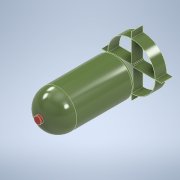
# Autodesk Inventor part: bomb
Saved by Autodesk Inventor 2022 (Build 260153000, 153)
## iProperties
Created: 2021-12-16
Part Number: bomb
Material: Generic
Document SubType Name: Modeling
Designer: jpc
Density: 1 g/cm^3
Appearance: Dark Olive
Author: jpc
Autodesk Inventor part; units mm, degrees
ref_plane "YZ Plane" through (0, 0, 0) normal (1, 0, 0) x (0, 1, 0)
ref_plane "XZ Plane" through (0, 0, 0) normal (0, 1, 0) x (-1, 0, 0)
ref_plane "XY Plane" through (0, 0, 0) normal (0, 0, 1) x (1, 0, 0)
sketch "Sketch1" plane through (0, 0, 0) normal (1, 0, 0) x (0, 1, 0)
  arc A0 (0, 250) -> (40, 251.6026) centre (0, 750) ccw
  line L0 (500, 750) -> (40, 750) construction
  line L1 (0, 750) -> (0, 250)
  line L2 (0, -750) -> (40, -750)
  line L3 (500, -750) -> (500, 750)
  line L4 (0, -750) -> (40, -750)
  line L5 (40, -750) -> (40, -1210) construction
  line L6 (40, -1500) -> (0, -1500)
  line L7 (0, -1500) -> (0, -750)
  line L8 (500, -750) -> (40, -1210)
  arc A1 (500, 750) -> (0, 1250) centre (0, 750) ccw
  arc A2 (0, 1250) -> (0, 250) centre (0, 750) ccw construction
  arc A3 (40, 251.6026) -> (500, 750) centre (0, 750) ccw construction
  line L9 (0, 250) -> (0, -750)
  line L10 (40, 750) -> (0, 750)
  line L11 (40, -750) -> (500, -750) construction
  line L12 (40, -1210) -> (40, -1500)
  line L13 (0, 1250) -> (0, 750)
  line L14 (500, 0) -> (0, 0)
  dimension "d1" = 1500
  dimension "d2" = 750
  dimension "d3" = 40
  dimension "d4" = 45
  dimension "d6" = 1000
  constraints: 30 end point, 9 parallel, 8 point on circle, 7 perpendicular, 4 centre point, 4 point on line, 3 horizontal, 2 coincident, 1 collinear, 1 midpoint
  measures "d1" distance of L3.start L0.start
  measures "d2" distance of L2.end L6.start
  measures "d3" distance of L6.start L6.end
  measures "d4" angle of L5 L8
  measures "d6" diameter of L3 L9
revolve "Revolution1" add sketch "Sketch1" angle 360 about axis through (0, 0, 250) along (0, 0, -1)
fillet "Fillet1" radius 75 2 edges at (0, -500, -750) (0, -40, -1210)
sketch "Sketch2" plane through (0, 0, 0) normal (0, 1, 0) x (-1, 0, 0)
  line L0 (-635, -1200) -> (-625, -1200)
  line L1 (-625, -1200) -> (-625, -1500)
  line L2 (-625, -1500) -> (-635, -1500)
  line L3 (-635, -1500) -> (-635, -1200)
  line L4 (-40, -1500) -> (40, -1500) projected
  line L5 (40, -1241.066) -> (-40, -1241.066) construction
  line L6 (-500, 750) -> (500, 750) projected
  line L7 (-500, -718.934) -> (500, -718.934) construction
  line L8 (0, -1241.066) -> (0, -1500)
  point P0 (0, 0)
  dimension "d8" = 258.934
  dimension "d9" = 300
  dimension "d10" = 1000
  dimension "d11" = 1250
  dimension "d12" = 80
  dimension "d13" = 10
  constraints: 10 end point, 2 midpoint, 2 parallel, 1 collinear, 1 horizontal, 1 perpendicular
  measures "d8" distance between parallel lines of L4 L5
  measures "d9" distance of L2.end L0.start
  measures "d10" distance of L7.start L7.end
  measures "d11" diameter of L1 L8
  measures "d12" distance of L4.start L4.end
  measures "d13" distance of L1.end L2.end
revolve "Revolution2" add sketch "Sketch2" angle 360 about axis through (0, 0, -1241.066) along (0, 0, -1)
sketch "Sketch3" plane through (0, 0, -1500) normal (0, 0, -1) x (-1, 0, 0)
  line L0 (793.75, 5) -> (-793.75, 5)
  line L1 (-793.75, 5) -> (-793.75, -5)
  line L2 (-793.75, -5) -> (793.75, -5)
  line L3 (793.75, -5) -> (793.75, 5)
  line L4 (793.75, 5) -> (-793.75, -5) construction
  circle A0 centre (0, 0) radius 635 construction
  circle A1 centre (0, 0) radius 625 construction
  line L5 (5, 793.75) -> (-5, 793.75)
  line L6 (-5, 793.75) -> (-5, -793.75)
  line L7 (-5, -793.75) -> (5, -793.75)
  line L8 (5, -793.75) -> (5, 793.75)
  line L9 (5, 793.75) -> (-5, -793.75) construction
  point P0 (0, 0)
  point P1 (0, 0)
  point P2 (5, -5)
  point P3 (5, 5)
  point P4 (-5, 5)
  point P5 (-5, -5)
  dimension "d15" = 1270
  dimension "d16" = 1250
  dimension "d17" = 10
  dimension "d18" = 1587.5
  dimension "d19" = 10
  dimension "d20" = 1587.5
  constraints: 20 end point, 4 parallel, 2 horizontal, 2 midpoint, 2 perpendicular, 1 coincident
  measures "d15" diameter of A0
  measures "d16" diameter of A1
  measures "d17" distance of L2.end L0.start
  measures "d18" distance of L1.end L2.end
  measures "d19" distance of L6.end L7.end
  measures "d20" distance of L5.end L6.end
extrude "Extrusion1" add sketch "Sketch3" against normal blind 300
sketch "Sketch5" plane through (0, 0, 0) normal (1, 0, 0) x (0, 1, 0)
  line L0 (793.75, -1200) -> (793.75, -1500) construction
  line L1 (793.75, -1500) -> (-793.75, -1500) construction
  line L2 (-793.75, -1500) -> (-793.75, -1200) construction
  line L3 (-61.967, -1188.033) -> (-478.033, -771.967) construction
  arc A0 (-500, -718.934) -> (-478.033, -771.967) centre (-425, -718.934) ccw construction
  line L4 (-500, -718.934) -> (-500, 750) construction
  arc A1 (0, 1250) -> (-500, 750) centre (0, 750) ccw construction
  arc A2 (500, 750) -> (0, 1250) centre (0, 750) ccw construction
  line L5 (500, 750) -> (500, -718.934) construction
  arc A3 (478.033, -771.967) -> (500, -718.934) centre (425, -718.934) ccw construction
  line L6 (478.033, -771.967) -> (61.967, -1188.033) construction
  line L7 (0, 750) -> (100, 750)
  line L8 (100, 750) -> (100, 1300)
  line L9 (100, 1300) -> (0, 1300)
  line L10 (0, 1300) -> (0, 750)
  line L11 (-793.75, -1200) -> (-52.2419, -1200) projected
  arc A4 (-52.2419, -1200) -> (-61.967, -1188.033) centre (-115, -1241.066) ccw projected
  arc A5 (61.967, -1188.033) -> (52.2419, -1200) centre (115, -1241.066) ccw projected
  line L12 (52.2419, -1200) -> (793.75, -1200) projected
  point P0 (0, 0)
  dimension "d28" = 500
  dimension "d29" = 550
  dimension "d30" = 100
  constraints: 8 end point, 2 parallel, 1 horizontal, 1 perpendicular
  measures "d28" radius of A2
  measures "d29" distance of L7.end L8.end
  measures "d30" distance of L8.end L9.end
revolve "Revolution4" add sketch "Sketch5" angle 360 about axis through (0, 0, 1300) along (0, 0, -1)
fillet "Face Fillet1" radius 10 1 edges at (0, -100, 1300)
sketch "Sketch6" plane through (0, 0, 0) normal (1, 0, 0) x (0, 1, 0)
  line L0 (793.75, -1300) -> (793.75, -1500) projected
  line L1 (793.75, -1500) -> (-793.75, -1500) construction
  line L2 (-793.75, -1500) -> (-793.75, -1300) construction
  line L3 (-61.967, -1188.033) -> (-478.033, -771.967) construction
  arc A0 (-500, -718.934) -> (-478.033, -771.967) centre (-425, -718.934) ccw construction
  line L4 (-500, -718.934) -> (-500, 750) construction
  arc A1 (-100, 1239.8979) -> (-500, 750) centre (0, 750) ccw construction
  line L5 (-100, 1239.8979) -> (-100, 1290) construction
  line L6 (100, 1290) -> (100, 1239.8979) construction
  arc A2 (500, 750) -> (100, 1239.8979) centre (0, 750) ccw construction
  line L7 (500, 750) -> (500, -718.934) construction
  arc A3 (478.033, -771.967) -> (500, -718.934) centre (425, -718.934) ccw construction
  line L8 (478.033, -771.967) -> (61.967, -1188.033) construction
  line L9 (500, 750) -> (500, -718.934) construction
  line L10 (500, 250) -> (505, 250)
  line L11 (505, 250) -> (505, -250)
  line L12 (505, -250) -> (500, -250)
  line L13 (500, -250) -> (500, 250)
  line L14 (500, -500) -> (505, -500)
  line L15 (505, -500) -> (505, -1000)
  line L16 (505, -1000) -> (500, -1000)
  line L17 (500, -1000) -> (500, -500)
  line L18 (500, 281.066) -> (505, 281.066)
  line L19 (505, 281.066) -> (505, -218.934)
  line L20 (505, -218.934) -> (500, -218.934)
  line L21 (500, -218.934) -> (500, 281.066)
  line L22 (0, -1762.2353) -> (0, 1823.4121) projected
  line L23 (-793.75, -1300) -> (-40, -1300) projected
  line L24 (40, -1300) -> (793.75, -1300) projected
  line L25 (-40, -1300) -> (-40, -1241.066) projected
  arc A4 (-40, -1241.066) -> (-61.967, -1188.033) centre (-115, -1241.066) ccw projected
  arc A5 (61.967, -1188.033) -> (40, -1241.066) centre (115, -1241.066) ccw projected
  line L26 (40, -1241.066) -> (40, -1300) projected
  arc A6 (-90, 1300) -> (-100, 1290) centre (-90, 1290) ccw projected
  line L27 (-90, 1300) -> (90, 1300) projected
  arc A7 (100, 1290) -> (90, 1300) centre (90, 1290) ccw projected
  point P0 (0, 0)
  dimension "d33" = 500
  dimension "d34" = 500
  dimension "d35" = 500
  dimension "d36" = 500
  dimension "d37" = 500
  dimension "d38" = 500
  dimension "d39" = 250
  dimension "d40" = 5
  constraints: 24 end point, 6 parallel, 5 point on line, 3 horizontal, 3 perpendicular
  measures "d33" radius of A2
  measures "d34" distance of L10.end L11.end
  measures "d35" distance of L14.end L15.end
  measures "d36" distance of L18.end L19.end
  measures "d37" distance from line of L20 A3.centre
  measures "d38" horizontal distance of L10.start A1.centre
  measures "d39" vertical distance of L14.end L12.end
  measures "d40" distance between parallel lines of L13 L11
equation "\"d2\" = 0.5 * d1"
equation "\"d3\" = 0.08 * d0"
equation "\"d11\" = 1.25 * d10"
equation "\"d13\" = 0.125 * d12"
equation "\"d17\" = -0.5 * d16 + 0.5 * d15"
equation "\"d18\" = 1.25 * d15"
equation "\"d19\" = d17"
equation "\"d20\" = d18"
equation "\"d29\" = 1.1 * d28"
equation "\"d30\" = 0.2 * d28"
equation "\"d34\" = d33"
equation "\"d35\" = d34"
equation "\"d36\" = d35"
equation "\"d37\" = d36"
equation "\"d38\" = d34"
equation "\"d39\" = 0.5 * d38"
equation "\"d40\" = 0.01 * d33"
equation "\"d0\" = 500"
body "Solid1"
body "Solid2"
